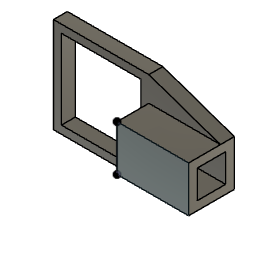
LightKnobExtender (Autodesk Fusion 360 design; units mm, degrees)
Autodesk Fusion 360 part; units mm, degrees
sketch "Sketch1" plane through (0, 0, 0) normal (0, 1, 0) x (1, 0, 0)
  line L0 (0, 0) -> (0, -11.5)
  line L1 (0, -11.5) -> (18, -11.5)
  line L2 (0, 0) -> (18, 0)
  line L3 (18, -11.5) -> (18, 0)
  dimension "d1" = 11.5
  dimension "d2" = 18
  dimension "d3" = 18
  constraint coincident L0.start L2.start
  constraint vertical L0
  constraint perpendicular L0 L1
  constraint perpendicular L0 L2
  measures "d1" distance of L0.start L0.end
  measures "d2" distance of L0.end L1.end
  measures "d3" distance of L0.start L2.end
extrude "Extrude1" add sketch "Sketch1" along normal blind 11.5
sketch "Sketch2" plane through (18, 0, 0) normal (1, 0, 0) x (0, 1, 0)
  line L0 (0, 11.5) -> (0, 0)
  line L1 (0, 0) -> (11.5, 0)
  line L2 (11.5, 0) -> (11.5, 11.5)
  line L3 (11.5, 11.5) -> (0, 11.5)
  line L4 (0, 11.5) -> (0, 9.3)
  line L5 (0, 9.3) -> (2.2, 9.3)
  line L6 (2.2, 9.3) -> (9.3, 9.3)
  line L7 (9.3, 9.3) -> (9.3, 2.2)
  line L8 (9.3, 2.2) -> (2.2, 2.2)
  line L9 (2.2, 2.2) -> (2.2, 9.3)
  dimension "d9" = 2.2
  dimension "d10" = 2.2
  dimension "d11" = 7.1
  dimension "d12" = 7.1
  constraint coincident L0.start L3.end
  constraint perpendicular L3 L4
  constraint perpendicular L4 L5
  constraint horizontal L6
  constraint vertical L7
  constraint horizontal L8
  constraint vertical L9
  measures "d9" distance of L0.start L4.end
  measures "d10" distance of L4.end L5.end
  measures "d11" distance of L5.end L6.end
  measures "d12" distance of L5.end L8.end
extrude "Extrude2" cut sketch "Sketch2" against normal blind 15 contours L6 L7 L8 L9
sketch "Sketch3" plane through (0, 0, 0) normal (-1, 0, 0) x (0, -1, 0)
  line L0 (0, 0) -> (0, 11.5)
  line L1 (0, 11.5) -> (-11.5, 11.5)
  line L2 (-11.5, 11.5) -> (-11.5, 0)
  line L3 (-11.5, 0) -> (0, 0)
  line L4 (-11.5, 11.5) -> (-7.25, 11.5)
  line L5 (-7.25, 11.5) -> (-7.25, 7.25)
  line L6 (-7.25, 7.25) -> (-4.25, 7.25)
  line L7 (-4.25, 7.25) -> (-4.25, 4.25)
  line L8 (-4.25, 4.25) -> (-7.25, 4.25)
  line L9 (-7.25, 4.25) -> (-7.25, 7.25)
  dimension "d15" = 4.25
  dimension "d16" = 4.25
  dimension "d17" = 3
  dimension "d18" = 3
  constraint coincident L1.end L2.start
  constraint perpendicular L2 L4
  constraint perpendicular L1 L5
  constraint horizontal L6
  constraint vertical L7
  constraint horizontal L8
  constraint vertical L9
  measures "d15" distance of L1.end L4.end
  measures "d16" distance of L4.end L5.end
  measures "d17" distance of L5.end L6.end
  measures "d18" distance of L5.end L8.end
sketch "Sketch4" plane through (0, 0, 0) normal (-1, 0, 0) x (0, -1, 0)
  line L0 (0, 0) -> (0, 11.5)
  line L1 (0, 11.5) -> (-11.5, 11.5)
  line L2 (-11.5, 11.5) -> (-11.5, 0)
  line L3 (-11.5, 0) -> (0, 0)
  line L4 (-11.5, 11.5) -> (-11.5, 7.5)
  line L5 (-11.5, 7.5) -> (0, 7.5)
  line L6 (0, 7.5) -> (0, 4)
  line L7 (0, 4) -> (-11.5, 4)
  line L8 (-11.5, 4) -> (-11.5, 7.5)
  dimension "d21" = 4
  dimension "d22" = 3.5
  constraint coincident L1.end L2.start
  constraint perpendicular L1 L4
  constraint horizontal L5
  constraint vertical L6
  constraint horizontal L7
  constraint vertical L8
  constraint coincident L0 L6.end
  measures "d21" distance of L1.end L4.end
  measures "d22" distance of L4.end L7.end
sketch "Sketch5" plane through (0, 0, 0) normal (0, -1, 0) x (1, 0, 0)
  line L0 (0, 11.5) -> (0, 0)
  line L1 (0, 0) -> (18, 0)
  line L2 (18, 0) -> (18, 11.5)
  line L3 (18, 11.5) -> (0, 11.5)
  line L4 (0, 11.5) -> (0, 0)
  constraint coincident L0.start L3.end
  constraint coincident L0.end L1.start
sketch "Sketch6" plane through (0, 11.5, 0) normal (0, 1, 0) x (-1, 0, 0)
  line L0 (0, 0) -> (0, 11.5)
  line L1 (0, 11.5) -> (-18, 11.5)
  line L2 (-18, 11.5) -> (-18, 0)
  line L3 (-18, 0) -> (0, 0)
  line L4 (0, 5.75) -> (24, 5.75)
  line L5 (24, 5.75) -> (24, 17.75)
  line L6 (24, 17.75) -> (0, 17.75)
  line L7 (0, 17.75) -> (0, 5.75)
  line L8 (0, 5.75) -> (-18, 5.75) construction
  line L9 (24, 5.75) -> (24, -6.25)
  line L10 (24, -6.25) -> (0, -6.25)
  line L11 (0, 5.75) -> (24, 5.75)
  line L12 (0, -6.25) -> (0, 0)
  dimension "d26" = 24
  dimension "d27" = 12
  constraint horizontal L4
  constraint vertical L5
  constraint horizontal L6
  constraint vertical L7
  constraint midpoint L0 L4.start
  constraint midpoint L2 L8.end
  constraint symmetric L4.start L8 L7.end
  constraint symmetric L4.end L8 L5.start
  constraint symmetric L5.end L8 L9.end
  constraint symmetric L6.end L8 L10.end
  constraint coincident L0.start L3.end
  measures "d26" distance of L4.start L4.end
  measures "d27" distance of L4.start L6.end
extrude "Extrude5" add sketch "Sketch6" against normal blind 3.5 contours L0 L4 L9 L10 L11 L12 | L0 L4 L5 L6 L7 L11
sketch "Sketch7" plane through (0, 11.5, 0) normal (0, 1, 0) x (-1, 0, 0)
  line L0 (0, 11.5) -> (-18, 11.5)
  line L1 (-18, 11.5) -> (-18, 0)
  line L2 (-18, 0) -> (0, 0)
  line L3 (0, 0) -> (0, -6.25)
  line L4 (0, -6.25) -> (24, -6.25)
  line L5 (24, -6.25) -> (24, 17.75)
  line L6 (24, 17.75) -> (0, 17.75)
  line L7 (0, 17.75) -> (0, 11.5)
  line L8 (24, -6.25) -> (24, -4.25)
  line L9 (24, -4.25) -> (22, -4.25)
  line L10 (22, -4.25) -> (2, -4.25)
  line L11 (2, -4.25) -> (2, 15.75)
  line L12 (2, 15.75) -> (22, 15.75)
  line L13 (22, 15.75) -> (22, -4.25)
  dimension "d30" = 2
  dimension "d31" = 2
  dimension "d32" = 20
  dimension "d33" = 20
  constraint coincident L4.end L5.start
  constraint perpendicular L4 L8
  constraint perpendicular L8 L9
  constraint horizontal L10
  constraint vertical L11
  constraint horizontal L12
  constraint vertical L13
  measures "d30" distance of L4.end L8.end
  measures "d31" distance of L8.end L9.end
  measures "d32" distance of L9.end L10.end
  measures "d33" distance of L9.end L12.end
extrude "Extrude6" cut sketch "Sketch7" against normal blind 5 contours L10 L11 L12 L13
sketch "Sketch8" plane through (0, 0, 0) normal (1, 0, 0) x (0, 1, 0)
sketch "Sketch9" plane through (0, 11.5, 0) normal (0, 1, 0) x (-1, 0, 0)
  line L0 (2, -4.25) -> (2, 15.75)
  line L1 (2, 15.75) -> (22, 15.75)
  line L2 (22, 15.75) -> (22, -4.25)
  line L3 (22, -4.25) -> (2, -4.25)
  line L4 (0, 11.5) -> (-18, 11.5)
  line L5 (-18, 11.5) -> (-18, 0)
  line L6 (-18, 0) -> (0, 0)
  line L7 (0, 0) -> (0, -6.25)
  line L8 (0, -6.25) -> (24, -6.25)
  line L9 (24, -6.25) -> (24, 17.75)
  line L10 (24, 17.75) -> (0, 17.75)
  line L11 (0, 17.75) -> (0, 11.5)
  line L12 (0, -6.25) -> (-18, 0)
  line L13 (0, 17.75) -> (-18, 11.5)
  constraint coincident L7.end L8.start
  constraint coincident L5.end L6.start
  constraint coincident L10.end L11.start
  constraint coincident L4.end L5.start
extrude "Extrude7" add sketch "Sketch9" against normal blind 3.5 contours L4 L11 L13 | L6 L7 L12
